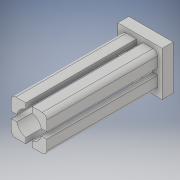
# Autodesk Inventor part: hjul-motor overgang different
Saved by Autodesk Inventor 2019 (Build 230136000, 136)
## iProperties
Created: 2019-03-12
Part Number: hjul-motor overgang different
Material: Generic
Document SubType Name: Modeling
Designer: jonas
Density: 1 g/cm^3
Appearance: Default
Author: jonas
Autodesk Inventor part; units mm, degrees
ref_plane "YZ Plane" through (0, 0, 0) normal (1, 0, 0) x (0, 1, 0)
ref_plane "XZ Plane" through (0, 0, 0) normal (0, 1, 0) x (-1, 0, 0)
ref_plane "XY Plane" through (0, 0, 0) normal (0, 0, 1) x (1, 0, 0)
sketch "Sketch1" plane through (0, 0, 0) normal (0, 0, 1) x (1, 0, 0)
  line L0 (-1.2, 1.6) -> (-0.2919, 1.6)
  line L1 (1.6, 1.2) -> (1.6, 0.2919)
  line L2 (1.2, -1.6) -> (0.2919, -1.6)
  line L3 (-1.6, -1.2) -> (-1.6, -0.2919)
  line L4 (0, -2.356) -> (0, 2.356) projected
  line L5 (-2.356, 0) -> (2.356, 0) projected
  arc A0 (-0.2919, 1.1123) -> (-1.1123, 0.2919) centre (0, 0) ccw
  line L6 (0.2919, 1.6) -> (0.2919, 1.1123)
  line L7 (0.2919, 1.6) -> (1.2, 1.6)
  line L8 (-0.2919, 1.1123) -> (-0.2919, 1.6)
  arc A1 (1.6, 1.2) -> (1.2, 1.6) centre (1.2, 1.2) ccw
  arc A2 (1.2, -1.6) -> (1.6, -1.2) centre (1.2, -1.2) ccw
  arc A3 (-1.6, -1.2) -> (-1.2, -1.6) centre (-1.2, -1.2) ccw
  arc A4 (-1.2, 1.6) -> (-1.6, 1.2) centre (-1.2, 1.2) ccw
  line L9 (-1.1123, -0.2919) -> (-1.6, -0.2919)
  line L10 (-1.6, 0.2919) -> (-1.1123, 0.2919)
  line L11 (0.2919, -1.1123) -> (0.2919, -1.6)
  line L12 (-0.2919, -1.6) -> (-0.2919, -1.1123)
  line L13 (1.1123, 0.2919) -> (1.6, 0.2919)
  line L14 (1.6, -0.2919) -> (1.1123, -0.2919)
  arc A5 (-1.1123, -0.2919) -> (-0.2919, -1.1123) centre (0, 0) ccw
  arc A6 (0.2919, -1.1123) -> (1.1123, -0.2919) centre (0, 0) ccw
  arc A7 (1.1123, 0.2919) -> (0.2919, 1.1123) centre (0, 0) ccw
  line L15 (1.6, -0.2919) -> (1.6, -1.2)
  line L16 (-0.2919, -1.6) -> (-1.2, -1.6)
  line L17 (-1.6, 0.2919) -> (-1.6, 1.2)
  dimension "d0" = 1.6
  dimension "d6" = 0.4
  dimension "d14" = 360
  constraints: 32 end point, 16 point on circle, 14 tangent, 9 parallel, 8 centre point, 4 perpendicular, 3 equal radius, 2 horizontal, 1 coincident, 27 other
  measures "d0" distance between parallel lines of L1 L4
  measures "d6" radius of A1
extrude "Extrusion3" add sketch "Sketch1" along normal blind 10
sketch "Sketch2" plane through (0, 0, 0) normal (0, 0, -1) x (-1, 0, 0)
  line L0 (2, 2) -> (-2, 2)
  line L1 (-2, 2) -> (-2, -2)
  line L2 (-2, -2) -> (2, -2)
  line L3 (2, -2) -> (2, 2)
  line L4 (2.8, 0) -> (-2.8, 0) projected
  line L5 (0, -2.8) -> (0, 2.8) projected
  circle A0 centre (0, 0) radius 1.15
  dimension "d18" = 4
  dimension "d19" = 4
  dimension "d22" = 2.3
  constraints: 8 end point, 2 parallel, 1 centre point, 1 coincident, 1 horizontal, 1 perpendicular, 2 other
  measures "d18" distance between parallel lines of L1 L3
  measures "d19" distance between parallel lines of L2 L0
  measures "d22" diameter of A0
extrude "Extrusion5" add sketch "Sketch2" along normal blind 1 contours L3 L4 A0 L5 L0 | L5 A0 L4 L1 L0 | L3 L2 L5 A0 L4 | L4 A0 L5 L2 L1
equation "\"d0\" = d1"
equation "\"d19\" = d18"
equation "\"d1\" = 1.6"
body "Solid3"
